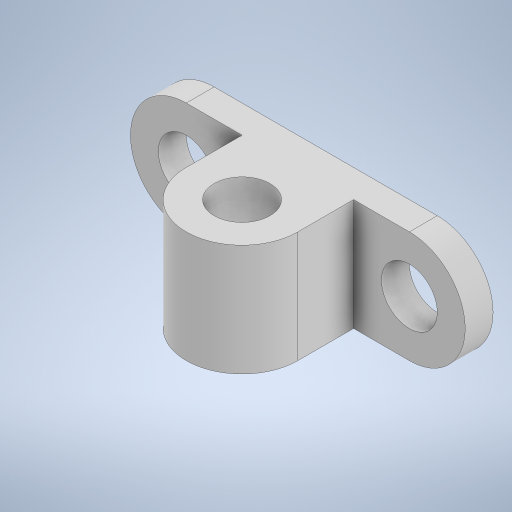
# Autodesk Inventor part: T1 - Darnnel Gonzalez
Saved by Autodesk Inventor 2024 (Build 280153000, 153)
## iProperties
Created: 2024-02-03
Part Number: T1 - Darnnel Gonzalez
Material: Generic
Document SubType Name: Modeling
Designer: darne
Density: 1 g/cm^3
Appearance: Default
Author: darne
Autodesk Inventor part; units mm, degrees
ref_plane "YZ Plane" through (0, 0, 0) normal (1, 0, 0) x (0, 1, 0)
ref_plane "XZ Plane" through (0, 0, 0) normal (0, 1, 0) x (-1, 0, 0)
ref_plane "XY Plane" through (0, 0, 0) normal (0, 0, 1) x (1, 0, 0)
sketch "Sketch1" plane through (0, 0, 0) normal (0, 0, 1) x (1, 0, 0)
  line L0 (-40, 20) -> (40, 20)
  line L1 (40, 20) -> (40, -20)
  line L2 (40, -20) -> (-40, -20)
  line L3 (-40, -20) -> (-40, 20)
  line L4 (-40, 20) -> (40, -20) construction
  line L5 (40, 20) -> (-40, -20) construction
  circle A0 centre (-40, 0) radius 10
  circle A1 centre (-40, 0) radius 20
  circle A2 centre (40, 0) radius 10
  circle A3 centre (40, 0) radius 20
  point P0 (0, 0)
  dimension "d0" = 80
  dimension "d1" = 40
  dimension "d2" = 20
  dimension "d3" = 40
  dimension "d4" = 20
  dimension "d5" = 40
  constraints: 12 end point, 4 centre point, 4 midpoint, 2 coincident, 2 parallel, 1 horizontal, 1 perpendicular
  measures "d0" distance of L1.end L2.end
  measures "d1" distance of L0.end L1.end
  measures "d2" diameter of A0
  measures "d3" diameter of A1
  measures "d4" diameter of A2
  measures "d5" diameter of A3
extrude "Extrusion1" add sketch "Sketch1" along normal blind 10
sketch "Sketch2" plane through (0, 0, 10) normal (0, 0, 1) x (1, 0, 0)
  arc A0 (-40, 20) -> (-40, -20) centre (-40, 0) ccw projected
  circle A1 centre (-40, 0) radius 10
  arc A2 (40, -20) -> (40, 20) centre (40, 0) ccw projected
  circle A3 centre (40, 0) radius 10
  line L0 (-20, -20) -> (20, -20)
  line L1 (20, -20) -> (20, 20)
  line L2 (20, 20) -> (-20, 20)
  line L3 (-20, 20) -> (-20, -20)
  line L4 (-20, -20) -> (20, 20) construction
  line L5 (20, -20) -> (-20, 20) construction
  point P0 (0, 0)
  dimension "d8" = 20
  dimension "d9" = 20
  dimension "d10" = 40
  dimension "d11" = 40
  constraints: 12 end point, 2 centre point, 2 coincident, 2 midpoint, 2 parallel, 1 horizontal, 1 perpendicular
  measures "d8" diameter of A1
  measures "d9" diameter of A3
  measures "d10" distance of L2.end L1.end
  measures "d11" distance of L1.end L0.end
extrude "Extrusion2" cut sketch "Sketch2" against normal blind 10 contours A1 | A3
sketch "Sketch3" plane through (0, 0, 10) normal (0, 0, 1) x (1, 0, 0)
  line L0 (-20, 20) -> (20, 20)
  line L1 (20, 20) -> (20, -20)
  line L2 (20, -20) -> (-20, -20)
  line L3 (-20, -20) -> (-20, 20)
  line L4 (-20, 20) -> (20, -20) construction
  line L5 (20, 20) -> (-20, -20) construction
  point P0 (0, 0)
  dimension "d14" = 40
  dimension "d15" = 40
  constraints: 12 end point, 2 midpoint, 2 parallel, 1 horizontal, 1 perpendicular
  measures "d14" distance of L1.end L2.end
  measures "d15" distance of L0.end L1.end
extrude "Extrusion3" add sketch "Sketch3" along normal blind 20
sketch "Sketch4" plane through (-40, -20, 0) normal (0, -1, 0) x (1, 0, 0)
  line L0 (60, 30) -> (20, 30) projected
  circle A0 centre (40, 30) radius 20
  point P0 (40, 0)
  dimension "d18" = 40
  constraints: 1 centre point, 1 midpoint
  measures "d18" diameter of A0
extrude "Extrusion4" add sketch "Sketch4" against normal blind 40 contours L0 A0 picked at (46.4729, 31.5954)
sketch "Sketch5" plane through (-40, 20, 0) normal (0, 1, 0) x (1, 0, 0)
  arc A0 (20, -30) -> (60, -30) centre (40, -30) ccw projected
  circle A1 centre (40, -30) radius 10
  point P0 (40, 0)
  dimension "d21" = 20
  constraints: 1 centre point, 1 coincident
  measures "d21" diameter of A1
extrude "Extrusion5" cut sketch "Sketch5" against normal blind 40
body "Solid1"
